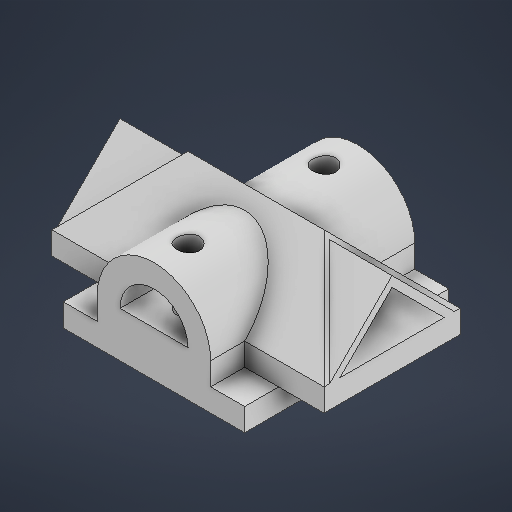
# Autodesk Inventor part: b4
Saved by Autodesk Inventor 2025.4 (Build 294407000, 407)
## iProperties
Created: 2026-05-15
Part Number: b4
Material: Generic
Document SubType Name: Modeling
Designer: VuQuan
Density: 1 g/cm^3
Appearance: Default
Author: VuQuan
Autodesk Inventor part; units mm, degrees
ref_plane "YZ Plane" through (0, 0, 0) normal (1, 0, 0) x (0, 1, 0)
ref_plane "XZ Plane" through (0, 0, 0) normal (0, 1, 0) x (-1, 0, 0)
ref_plane "XY Plane" through (0, 0, 0) normal (0, 0, 1) x (1, 0, 0)
sketch "Sketch1" plane through (0, 0, 0) normal (0, 0, 1) x (1, 0, 0)
  line L0 (0, 0) -> (-40, 0)
  line L1 (-40, 0) -> (-40, 10)
  line L2 (-40, 10) -> (-25, 10)
  line L3 (-25, 10) -> (-25, 20)
  arc A0 (0, 45) -> (-25, 20) centre (0, 20) ccw
  line L4 (0, 0) -> (0, 45) construction
  line L5 (0, 0) -> (40, 0)
  line L6 (40, 0) -> (40, 10)
  line L7 (40, 10) -> (25, 10)
  line L8 (25, 10) -> (25, 20)
  arc A1 (25, 20) -> (0, 45) centre (0, 20) ccw
  arc A2 (15, 20) -> (-15, 20) centre (0, 20) ccw
  line L9 (15, 20) -> (-15, 20)
  dimension "d0" = 10
  dimension "d1" = 25
  dimension "d2" = 80
  dimension "d3" = 10
  dimension "d4" = 15
  constraints: 20 end point, 6 point on circle, 4 symmetric about line, 3 centre point, 3 perpendicular, 2 horizontal, 2 horizontal alignment, 1 coincident, 1 point on line, 1 tangent, 1 vertical, 1 other
  measures "d0" distance of L0.end L1.end
  measures "d1" radius of A0
  measures "d2" diameter of L1 L4
  measures "d3" distance of L2.end L3.end
  measures "d4" radius of A2
extrude "Extrusion1" add sketch "Sketch1" along normal mid plane 90 contours L0 L1 L2 L3 A0 A1 L8 L7 L6 L5 | L9 A2
sketch "Sketch2" plane through (0, 0, 0) normal (1, 0, 0) x (0, 1, 0)
  line L0 (20, -30) -> (20, -27.5)
  line L1 (20, 30) -> (50, 0)
  line L2 (50, 0) -> (20, -30)
  line L3 (20, -30) -> (10, -30)
  line L4 (10, -30) -> (10, 30)
  line L5 (10, 30) -> (20, 30)
  line L6 (20, -27.5) -> (47.5, 0)
  line L7 (47.5, 0) -> (20, 27.5)
  line L8 (20, 27.5) -> (20, 30)
  line L9 (20, -27.5) -> (20, 27.5)
  point P0 (0, 0)
  point P1 (20, 0)
  dimension "d7" = 10
  dimension "d8" = 20
  dimension "d9" = 60
  dimension "d10" = 50
  dimension "d11" = 55
  constraints: 20 end point, 3 horizontal alignment, 3 perpendicular, 3 vertical, 2 horizontal, 1 parallel
  measures "d7" distance of L4.end L1.start
  measures "d8" distance from line of point (0, 0) L0
  measures "d9" distance of L3.end L4.end
  measures "d10" distance of point (0, 0) L1.end
  measures "d11" distance of L0.end L7.end
extrude "Extrusion2" add sketch "Sketch2" along normal mid plane 120
sketch "Sketch3" plane through (-60, 20, 30) normal (0, 0, 1) x (1, 0, 0)
  line L0 (0, 30) -> (120, 30) projected
  line L1 (0, 0) -> (0, 30) projected
  line L2 (30, 30) -> (0, 0)
  point P0 (60, -20)
  dimension "d16" = 30
  constraints: 2 end point, 1 point on line
  measures "d16" distance from line of L1 L2.start
extrude "Extrusion4" cut sketch "Sketch3" along normal through all both and the other way through all
mirror "Mirror2" about plane through (0, 0, 0) normal (1, 0, 0) of "Extrusion4"
extrude "Extrusion5" add sketch "Sketch2" along normal mid plane 120 contours L9 L7 L6
sketch "Sketch4" plane through (-60, 0, 0) normal (-1, 0, 0) x (0, 0, 1)
  line L0 (0, 47.5) -> (-27.5, 20) projected
  line L1 (-27.5, 20) -> (-30, 20) projected
  line L2 (0, 43) -> (-23, 20)
  line L3 (-23, 20) -> (23, 20)
  line L4 (23, 20) -> (0, 43)
  point P0 (0, 0)
  dimension "d21" = 43
  constraints: 6 end point, 1 collinear, 1 horizontal, 1 parallel, 1 perpendicular, 1 vertical alignment
  measures "d21" distance of L2.start point (0, 0)
extrude "Extrusion6" cut sketch "Sketch4" along normal up to surface surface through (-60, 20, 30) normal (0.7071068, -0.7071068, 0)
mirror "Mirror3" about plane through (0, 0, 0) normal (1, 0, 0) of "Extrusion6"
extrude "Extrusion3" cut sketch "Sketch1" along normal through all both and the other way through all contours L9 A2
sketch "Sketch5" plane through (-40, 0, 45) normal (0, -1, 0) x (1, 0, 0)
  circle A0 centre (40, -15) radius 5
  line L0 (80, -15) -> (100, -15) projected
  circle A1 centre (40, -75) radius 5
  line L1 (80, -75) -> (100, -75) projected
  point P0 (40, -45)
  dimension "d24" = 10
  constraints: 2 centre point, 2 point on line, 2 vertical alignment, 1 equal radius
  measures "d24" diameter of A0
extrude "Extrusion7" cut sketch "Sketch5" against normal through all
body "Solid1"
